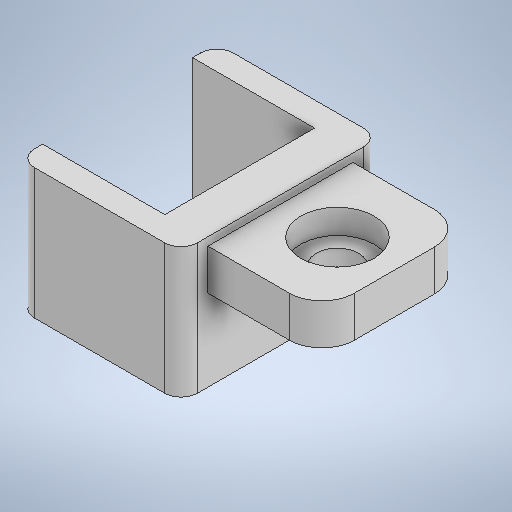
# Autodesk Inventor part: input_holder
Saved by Autodesk Inventor 2025 (Build 290162000, 162)
## iProperties
Created: 2026-05-15
Part Number: input_holder
Material: Ogólny
Document SubType Name: Modeling
Designer: zzapa
Density: 1 g/cm^3
Appearance: Domyślna
Author: zzapa
Autodesk Inventor part; units mm, degrees
ref_plane "YZ Plane" through (0, 0, 0) normal (1, 0, 0) x (0, 1, 0)
ref_plane "XZ Plane" through (0, 0, 0) normal (0, 1, 0) x (-1, 0, 0)
ref_plane "XY Plane" through (0, 0, 0) normal (0, 0, 1) x (1, 0, 0)
sketch "Szkic1" plane through (0, 0, 0) normal (0, 1, 0) x (-1, 0, 0)
  line L0 (2.5, 6.1) -> (0, 6.1)
  line L1 (0, 6.1) -> (0, -6.1)
  line L2 (0, -6.1) -> (2.5, -6.1)
  line L3 (2.5, -6.1) -> (2.5, 6.1)
  line L4 (0, 6.1) -> (10, 6.1)
  line L5 (10, 6.1) -> (10, 4.6)
  line L6 (10, 4.6) -> (0, 4.6)
  line L7 (0, 4.6) -> (0, 6.1)
  line L8 (0, -4.6) -> (10, -4.6)
  line L9 (10, -4.6) -> (10, -6.1)
  line L10 (10, -6.1) -> (0, -6.1)
  line L11 (0, -6.1) -> (0, -4.6)
  point P0 (0, 0)
  point P1 (0, 0)
  point P2 (2.5, -6.1)
  point P3 (2.5, -4.6)
  point P4 (2.5, 4.6)
  dimension "d0" = 2.5
  dimension "d1" = 9.2
  dimension "d2" = 10
  dimension "d3" = 1.5
  dimension "d4" = 1.5
  constraints: 24 end point, 6 parallel, 4 collinear, 3 horizontal, 3 perpendicular, 1 coincident, 1 midpoint, 1 point on line
  measures "d0" distance between parallel lines of L1 L3
  measures "d1" distance between parallel lines of L8 L6
  measures "d2" distance between parallel lines of L1 L5
  measures "d3" distance between parallel lines of L10 L8
  measures "d4" distance between parallel lines of L6 L4
extrude "Wyciągnięcie proste1" add sketch "Szkic1" along normal blind 8
ref_plane "Płaszczyzna konstrukcyjna1" through (0, 5, 0) normal (0, -1, 0) x (1, 0, 0)
sketch "Szkic2" plane through (0, 5, 0) normal (0, -1, 0) x (1, 0, 0)
  line L0 (7, -4.45) -> (0, -4.45)
  line L1 (0, -4.45) -> (0, 4.45)
  line L2 (0, 4.45) -> (7, 4.45)
  line L3 (7, 4.45) -> (7, -4.45)
  point P0 (0, 0)
  point P1 (0, 0)
  dimension "d8" = 8.9
  dimension "d9" = 7
  constraints: 8 end point, 2 parallel, 1 coincident, 1 horizontal, 1 midpoint, 1 perpendicular
  measures "d8" distance of L2.end L0.start
  measures "d9" distance of L0.start L0.end
extrude "Wyciągnięcie proste2" add sketch "Szkic2" against normal blind 2.5
sketch "Szkic3" plane through (0, 7.5, 0) normal (0, 1, 0) x (1, 0, 0)
  line L0 (3.5, -4) -> (3.5, 4)
  line L1 (-13.4, 0) -> (10.4, 0) projected
  line L2 (7, 4.45) -> (0, 4.45) projected
  line L3 (0, -4.45) -> (7, -4.45) projected
  point P0 (0, 0)
  point P1 (3.5, 0)
  point P2 (0, 4.45)
  point P3 (3.5, -4.45)
  point P4 (3.5, 4.45)
  constraints: 2 end point, 1 midpoint, 1 point on line, 6 other
hole "Otwór1" at (3.5, 7.5, 0) direction (0, -1, 0) diameter 2.6 end through all counterbore diameter 4.5 counterbore depth 1.5
fillet "Zaokrąglenie1" radius 2 2 edges at (7, 6.25, 4.45) (7, 6.25, -4.45)
fillet "Zaokrąglenie2" radius 1 4 edges at (-10, 4, -6.1) (0, 4, -6.1) (-10, 4, 6.1) (0, 4, 6.1)
equation "\"d0\" = holder_gniazdo_grubosc"
equation "\"d1\" = holder_gniazdo_odleglosc_miedzy_ramionami"
equation "\"d2\" = holder_gniazdo_dlugosc_ramion"
equation "\"d3\" = holder_gniazdo_grubosc_ramion"
equation "\"d4\" = holder_gniazdo_grubosc_ramion"
equation "\"d5\" = holder_gniazdo_wys"
equation "\"d8\" = podstawa_mocowanie_DC_b"
equation "\"d9\" = podstawa_mocowanie_DC_a"
equation "\"d10\" = holder_gniazdo_grubosc"
equation "\"d12\" = gniazdo_M2_D2"
equation "\"d14\" = gniazdo_M2_D1"
equation "\"d15\" = gniazdo_M2_glebokosc"
equation "\"gniazdo_M2_glebokosc\" = 1.5"
equation "\"gniazdo_M2_D1\" = 4.5"
equation "\"gniazdo_M2_D2\" = 2.6"
equation "\"insert_D\" = 2.9"
equation "\"insert_glebokosc\" = 7"
equation "\"podstawa_wys\" = 2"
equation "\"podstawa_otwory_montazowe_poz_x\" = 4"
equation "\"podstawa_otwory_montazowe_poz_y\" = 4"
equation "\"podstawa_zaokraglenie\" = 3"
equation "\"obudowa_wys\" = 45"
equation "\"obudowa_grubosc\" = 2"
equation "\"obudowa_kontrolki_a\" = 38"
equation "\"obudowa_otwory_montazowe_poz_x\" = 4"
equation "\"obudowa_otwory_montazowe_poz_y\" = 4"
equation "\"obudowa_otwory_montazowe_material_x\" = 8"
equation "\"obudowa_otwory_montazowe_material_y\" = 8"
equation "\"obudowa_zaokraglenie\" = 3"
equation "\"obudowa_otwory_io1_D\" = 12"
equation "\"obudowa_otwory_io1_wys\" = 25"
equation "\"obudowa_otwory_io1_poz\" = 55"
equation "\"obudowa_otwory_io2_D\" = 12"
equation "\"obudowa_otwory_io2_wys\" = 25"
equation "\"obudowa_otwory_io2_poz\" = 38"
equation "\"obudowa_otwory_pot_D\" = 7.2"
equation "\"obudowa_pot_poz_y\" = 15"
equation "\"obudowa_s_rozstaw_y\" = 16"
equation "\"obudowa_s_poz_x\" = 78"
equation "\"obudowa_s_poz_y\" = 15"
equation "\"obudowa_s_D\" = 6.2"
equation "\"input_a\" = 8.9"
equation "\"input_b\" = 14.4"
equation "\"input_wys\" = 10.9"
equation "\"obudowa_MTS_otwor_D\" = 6.2"
equation "\"pcb_rozstaw_x\" = 92"
equation "\"pcb_rozstaw_y\" = 58"
equation "\"pcb_grubosc_scianki\" = 6"
equation "\"pcb_wys_bloku\" = 35"
equation "\"pcb_poz_y\" = 29"
equation "\"obudowa_footswitch_D\" = 12.3"
equation "\"obudowa_footswitch_poz_x\" = 35"
equation "\"obudowa_footswitch_poz_y\" = 68"
equation "\"obudowa_led_indicator_D\" = 3.5"
equation "\"obudowa_led_indicator_poz_x\" = 55"
equation "\"obudowa_podkladka_otwory\" = 4"
equation "\"obudowa_uchwyt_poz_z\" = 3"
equation "\"obudowa_uchwyt_grubosc\" = 2"
equation "\"obudowa_uchwyt_szerokosc_wew\" = 17.5"
equation "\"obudowa_uchwyt_wysokosc_wew\" = 26.3"
equation "\"obudowa_uchwyt_kolnierz_wys\" = 55"
equation "\"obudowa_gniazdo_poz\" = 25"
equation "\"obudowa_podciecie_inout_wys\" = 6"
equation "\"obudowa_podciecie_logo_wys\" = 34"
equation "\"obudowa_podciecie_logo_szerokosc\" = 25"
equation "\"obudowa_pot_pozycjonowanie_szerokosc\" = 2.8"
equation "\"obudowa_pot_pozycjonowanie_wys\" = 13"
equation "\"obudowa_pot_pozycjonowanie_glebokosc\" = 1.4"
equation "\"obudowa_led_mocowanie_wys\" = 6"
equation "\"obudowa_led_mocowanie_grubosc\" = 8"
equation "\"holder_led_grubosc\" = 2.5"
equation "\"holder_led_dlugosc\" = 28"
equation "\"holder_led_uchwyt_D\" = 5"
equation "\"holder_led_uchwyt_szerokosc\" = 8"
equation "\"holder_led_uchwyt_wysokosc\" = 5"
equation "\"holder_gniazdo_grubosc\" = 2.5"
equation "\"holder_gniazdo_a\" = 28"
equation "\"holder_gniazdo_b\" = 5"
equation "\"podstawa_mocowanie_DC_a\" = 7"
equation "\"podstawa_mocowanie_DC_b\" = 8.9"
equation "\"podstawa_mocowanie_DC_wys\" = 6"
equation "\"holder_gniazdo_odleglosc_miedzy_ramionami\" = 9.2"
equation "\"holder_gniazdo_dlugosc_ramion\" = 10"
equation "\"holder_gniazdo_grubosc_ramion\" = 1.5"
equation "\"holder_gniazdo_wys\" = 8"
equation "\"holder_gniazdo_uchwyt_poz\" = 5"
equation "\"d7\" = -holder_gniazdo_uchwyt_poz"
